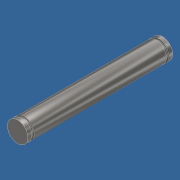
# Autodesk Inventor part: AxeVerticalCaptif
Saved by Autodesk Inventor 2018 (Build 220112000, 112)
## iProperties
Created: 2022-03-25
Part Number: AxeVerticalCaptif
Material: Stainless Steel
Document SubType Name: Modeling
Designer: Nathann
Density: 8 g/cm^3
Appearance: Semi-Polished
Mass: 21.4681 g
Surface Area: 17.1052 cm^2
Volume: 2.68352 cm^3
Author: Nathann
Autodesk Inventor part; units mm, degrees
ref_plane "XZ Plane" through (0, 0, 0) normal (0, 1, 0) x (-1, 0, 0)
ref_plane "XY Plane" through (0, 0, 0) normal (0, 0, 1) x (1, 0, 0)
sketch "Sketch1" plane through (0, 0, 0) normal (0, 1, 0) x (-1, 0, 0)
  arc A0 (3.873, 1) -> (3.873, -1) centre (0, 0) ccw
  circle A1 centre (0, 0) radius 4
  dimension "d0" = 8
  constraints: 2 coincident, 2 point on circle, 1 centre point, 3 other
  measures "d0" diameter of A0
extrude "Extrusion1" add sketch "Sketch1" along normal blind 56.5
sketch "Sketch2" plane through (0, 0, 0) normal (1, 0, 0) x (0, 1, 0)
  line L0 (1.5, -6.5) -> (2.44, -6.5)
  line L1 (2.44, -6.5) -> (2.44, -3.5)
  line L2 (2.44, -3.5) -> (1.5, -3.5)
  line L3 (1.5, -3.5) -> (1.5, -6.5)
  line L4 (0, -4) -> (56.5, -4) projected
  line L5 (0, -4) -> (56.5, -4) projected
  line L6 (0, -4) -> (56.5, -4) projected
  line L7 (0, -4) -> (0, 4) projected
  line L8 (28.25, -4) -> (28.25, 9.3026)
  line L9 (55, -6.5) -> (54.06, -6.5)
  line L10 (54.06, -6.5) -> (54.06, -3.5)
  line L11 (54.06, -3.5) -> (55, -3.5)
  line L12 (55, -3.5) -> (55, -6.5)
  line L13 (56.5, -4) -> (56.5, 4)
  line L14 (-11.3, 0) -> (67.8, 0) projected
  point P0 (0, 0)
  point P1 (0, 1)
  point P2 (0, -1)
  point P3 (56.5, 0)
  point P4 (56.5, 1)
  point P5 (56.5, -1)
  dimension "d9" = 0.94
  dimension "d10" = 0.5
  dimension "d11" = 3
  dimension "d12" = 1.5
  constraints: 20 end point, 11 symmetric about line, 2 parallel, 1 horizontal, 1 midpoint, 1 perpendicular, 1 vertical
  measures "d9" distance between parallel lines of L3 L1
  measures "d10" distance between parallel lines of L4 L2
  measures "d11" distance of L2.end L0.start
  measures "d12" distance between parallel lines of L7 L3
revolve "Revolution1" cut sketch "Sketch2" angle 360 about axis through (0, -10, 0) along (0, 1, 0) contours L3 L4 L1 L0 | L3 L2 L1 L4 | L10 L11 L12 L4 | L4 L12 L9 L10
ref_plane "Work Plane1" through (-4, 0, 0) normal (1, 0, 0) x (0, 1, 0)
sketch "Sketch5" plane through (-4, 0, 0) normal (1, 0, 0) x (0, 1, 0)
  line L0 (42.5, 1) -> (24.5, 1)
  line L1 (24.5, 1) -> (24.5, -1)
  line L2 (24.5, -1) -> (42.5, -1)
  line L3 (42.5, -1) -> (42.5, 1)
  circle A0 centre (24.5, 0) radius 1
  circle A1 centre (42.5, 0) radius 1
  line L4 (2.44, -4) -> (54.06, -4) projected
  line L5 (2.44, 4) -> (54.06, 4) projected
  line L6 (56.5, -4) -> (56.5, 4) projected
  line L7 (0, 4) -> (0, -4) projected
  point P0 (0, 0)
  dimension "d19" = 2
  dimension "d20" = 3
  dimension "d23" = 18
  dimension "d25" = 14
  constraints: 8 end point, 2 midpoint, 2 parallel, 2 vertical alignment, 1 horizontal, 1 perpendicular, 4 other
  measures "d19" distance between parallel lines of L0 L2
  measures "d20" distance between parallel lines of L2 L4
  measures "d23" distance of point (24.5, 0) point (42.5, 0)
  measures "d25" distance from line of L6 point (42.5, 0)
extrude "Extrusion4" cut sketch "Sketch5" along normal blind 1.2
body "Solid1"
